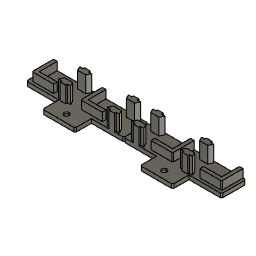
WT#LXLX R+L (Autodesk Fusion 360 design; units mm, degrees)
Autodesk Fusion 360 part; units mm, degrees
note: some values were not read from the file. Set by a fixed rule: which sketch regions a step uses.
sketch "Sketch1" plane through (0, 0, 0) normal (0, 0, 1) x (1, 0, 0)
  line L0 (90, 0) -> (90, 30)
  line L1 (90, 30) -> (0, 30)
  line L2 (0, 30) -> (0, 0)
  line L3 (15, 30) -> (11.5, 30)
  line L4 (15, 30) -> (18.5, 30)
  line L5 (18.5, 30) -> (18.5, 28)
  line L6 (18.5, 28) -> (22.5, 28)
  line L7 (11.5, 30) -> (11.5, 28)
  line L8 (11.5, 28) -> (7.5, 28)
  line L9 (15, 23) -> (20, 23)
  line L10 (15, 23) -> (10, 23)
  line L11 (10, 23) -> (7.5, 28)
  line L12 (20, 23) -> (22.5, 28)
  line L13 (15, 7) -> (10, 7)
  line L14 (15, 7) -> (20, 7)
  line L15 (15, 0) -> (18.5, 0)
  line L16 (18.5, 0) -> (18.5, 2)
  line L17 (18.5, 2) -> (22.5, 2)
  line L18 (22.5, 2) -> (20, 7)
  line L19 (15, 0) -> (11.5, 0)
  line L20 (11.5, 0) -> (11.5, 2)
  line L21 (11.5, 2) -> (7.5, 2)
  line L22 (7.5, 2) -> (10, 7)
  line L23 (75, 30) -> (71.5, 30)
  line L24 (75, 30) -> (78.5, 30)
  line L25 (75, 23) -> (70, 23)
  line L26 (75, 23) -> (80, 23)
  line L27 (78.5, 30) -> (78.5, 28)
  line L28 (78.5, 28) -> (82.5, 28)
  line L29 (82.5, 28) -> (80, 23)
  line L30 (71.5, 30) -> (71.5, 28)
  line L31 (71.5, 28) -> (67.5, 28)
  line L32 (67.5, 28) -> (70, 23)
  line L33 (75, 0) -> (71.5, 0)
  line L34 (75, 7) -> (70, 7)
  line L35 (75, 7) -> (80, 7)
  line L36 (71.5, 0) -> (71.5, 2)
  line L37 (71.5, 2) -> (67.5, 2)
  line L38 (67.5, 2) -> (70, 7)
  line L39 (75, 0) -> (78.5, 0)
  line L40 (78.5, 0) -> (78.5, 2)
  line L41 (78.5, 2) -> (82.5, 2)
  line L42 (82.5, 2) -> (80, 7)
  line L43 (0, 15) -> (30, 15)
  line L44 (30, 30) -> (30, 0)
  line L45 (60, 30) -> (60, 0)
  line L46 (0, 0) -> (30, 0)
  line L47 (30, 0) -> (60, 0)
  line L48 (60, 0) -> (90, 0)
  line L49 (30, 3.5) -> (56.5, 3.5)
  line L50 (56.5, 30) -> (56.5, 3.5)
  line L51 (52, 30) -> (52, 8)
  line L52 (30, 8) -> (52, 8)
  dimension "d1" = 30
  dimension "d2" = 90
  dimension "d8" = 3.5
  dimension "d9" = 7
  dimension "d13" = 7
  dimension "d19" = 4
  dimension "d21" = 3.5
  dimension "d22" = 7
  dimension "d26" = 4
  dimension "d27" = 4
  dimension "d28" = 7
  dimension "d29" = 3.5
  dimension "d35" = 30
  dimension "d38" = 3.5
  dimension "d39" = -8
  constraint vertical L0
  constraint horizontal L1
  constraint vertical L2
  constraint coincident L2.end L46.start
  constraint coincident L1 L3.start
  constraint perpendicular L4 L5
  constraint perpendicular L5 L6
  constraint perpendicular L3 L7
  constraint perpendicular L15 L16
  constraint perpendicular L16 L17
  constraint perpendicular L19 L20
  constraint perpendicular L20 L21
  constraint coincident L1 L23.start
  constraint parallel L1 L24
  constraint perpendicular L1 L27
  constraint perpendicular L27 L28
  constraint perpendicular L1 L30
  constraint perpendicular L30 L31
  constraint perpendicular L36 L37
  constraint perpendicular L39 L40
  constraint perpendicular L40 L41
  constraint midpoint L2 L43.start
  constraint perpendicular L2 L43
  constraint coincident L1 L44.start
  constraint coincident L1 L45.start
  constraint perpendicular L0 L46
  constraint perpendicular L45 L47
  constraint perpendicular L0 L48
  measures "d1" distance of L2.end L1.end
  measures "d2" distance of L2.end L0.start
  measures "d8" distance of L3.start L4.end
  measures "d9" distance of L3.start L9.start
  measures "d13" distance of L15.start L13.start
  measures "d19" distance of L20.end L21.end
  measures "d21" distance of L23.start L24.end
  measures "d22" distance of L23.start L25.start
  measures "d26" distance of L27.end L28.end
  measures "d27" distance of L30.end L31.end
  measures "d28" distance of L33.start L34.start
  measures "d29" distance of L33.start L33.end
  measures "d35" distance of L43.start L43.end
  measures "d59" distance of L2.end
  measures "d63" diameter of L2.end
extrude "Extrude1" add sketch "Sketch1" against normal blind 5 makes body 1
extrude "Extrude2" add sketch "Sketch1" along normal blind 20 contours L33 L34 L35 L36 L37 L38 L39 L40 L41 L42 L48 | L1 L23 L24 L25 L26 L27 L28 L29 L30 L31 L32 | L13 L14 L15 L16 L17 L18 L19 L20 L21 L22 L46 | L1 L3 L4 L5 L6 L7 L8 L9 L10 L11 L12 bodies 1
extrude "Extrude3" add sketch "Sketch1" along normal blind 10 contours L1 L44 L49 L50 L51 L52 bodies 1
chamfer "Chamfer1" distance 1.5 angle 45 4 edges at (90, 0, -2.5) (90, 30, -2.5) (0, 0, -2.5) (0, 30, -2.5) on bodies 1
chamfer "Chamfer2" distance 1 angle 45 1 edges at (56.5, 3.5, 5) on bodies 1
delete_face "DeleteFace1" 1 faces at (89.5, 1, -1.6667) on bodies 1
delete_face "DeleteFace2" 1 faces at (89, 29.5, -3.3333) on bodies 1
extrude "Extrude4" add 1 faces at (90, 10, -1.6667) along direction (1, 0, 0) blind 30 on bodies 1 bodies 1
sketch "Sketch2" plane through (0, 0, 0) normal (0, 0, 1) x (-1, 0, 0)
  line L0 (-120, -30) -> (-78.5, -30)
  line L1 (-78.5, -30) -> (-78.5, -28)
  line L2 (-78.5, -28) -> (-82.5, -28)
  line L3 (-82.5, -28) -> (-80, -23)
  line L4 (-80, -23) -> (-70, -23)
  line L5 (-70, -23) -> (-67.5, -28)
  line L6 (-67.5, -28) -> (-71.5, -28)
  line L7 (-71.5, -28) -> (-71.5, -30)
  line L8 (-71.5, -30) -> (-56.5, -30)
  line L9 (-56.5, -30) -> (-56.5, -4.5)
  line L10 (-56.5, -4.5) -> (-55.5, -3.5)
  line L11 (-55.5, -3.5) -> (-30, -3.5)
  line L12 (-30, -3.5) -> (-30, -8)
  line L13 (-30, -8) -> (-52, -8)
  line L14 (-52, -8) -> (-52, -30)
  line L15 (-52, -30) -> (-18.5, -30)
  line L16 (-18.5, -30) -> (-18.5, -28)
  line L17 (-18.5, -28) -> (-22.5, -28)
  line L18 (-22.5, -28) -> (-20, -23)
  line L19 (-20, -23) -> (-10, -23)
  line L20 (-10, -23) -> (-7.5, -28)
  line L21 (-7.5, -28) -> (-11.5, -28)
  line L22 (-11.5, -28) -> (-11.5, -30)
  line L23 (-11.5, -30) -> (-1.5, -30)
  line L24 (-1.5, -30) -> (0, -28.5)
  line L25 (0, -28.5) -> (0, -1.5)
  line L26 (0, -1.5) -> (-1.5, 0)
  line L27 (-1.5, 0) -> (-11.5, 0)
  line L28 (-11.5, 0) -> (-11.5, -2)
  line L29 (-11.5, -2) -> (-7.5, -2)
  line L30 (-7.5, -2) -> (-10, -7)
  line L31 (-10, -7) -> (-20, -7)
  line L32 (-20, -7) -> (-22.5, -2)
  line L33 (-22.5, -2) -> (-18.5, -2)
  line L34 (-18.5, -2) -> (-18.5, 0)
  line L35 (-18.5, 0) -> (-71.5, 0)
  line L36 (-71.5, 0) -> (-71.5, -2)
  line L37 (-71.5, -2) -> (-67.5, -2)
  line L38 (-67.5, -2) -> (-70, -7)
  line L39 (-70, -7) -> (-80, -7)
  line L40 (-80, -7) -> (-82.5, -2)
  line L41 (-82.5, -2) -> (-78.5, -2)
  line L42 (-78.5, -2) -> (-78.5, 0)
  line L43 (-78.5, 0) -> (-120, 0)
  line L44 (-120, 0) -> (-120, -30)
  line L45 (-120, 0) -> (-90, 0)
  line L46 (-120, 0) -> (-120, -30)
  line L47 (-116.5, -3.5) -> (-90, -3.5)
  line L48 (-116.5, -3.5) -> (-116.5, -30)
  line L49 (-112, -8) -> (-112, -30)
  line L50 (-112, -8) -> (-90, -8)
  line L51 (-90, -3.5) -> (-90, -8)
  dimension "d50" = 30
  dimension "d51" = -3.5
  dimension "d52" = 8
  constraint coincident L43.end L44.start
  constraint perpendicular L44 L45
  constraint coincident L0.start L44.end
  constraint perpendicular L50 L51
  measures "d50" distance of L43.end L45.end
extrude "Extrude5" add sketch "Sketch2" along normal blind 10 contours L0 L47 L48 L49 L50 L51 bodies 1
chamfer "Chamfer3" distance 1 angle 45 1 edges at (116.5, 3.5, 5) on bodies 1
chamfer "Chamfer4" distance 1.5 angle 45 2 edges at (120, 0, -2.5) (120, 30, -2.5) on bodies 1
mirror "Mirror1" about plane through (0, 0, 0) normal (1, 0, 0) of bodies 1 makes body 2
sketch "Sketch3" plane through (0, 0, 0) normal (0, -1, 0) x (1, 0, 0)
  line L0 (-118.5, 0) -> (-118.5, -5)
  line L1 (-118.5, -5) -> (-1.5, -5)
  line L2 (-1.5, -5) -> (-1.5, 0)
  line L3 (-1.5, 0) -> (-11.5, 0)
  line L4 (-11.5, 0) -> (-11.5, 20)
  line L5 (-11.5, 20) -> (-18.5, 20)
  line L6 (-18.5, 20) -> (-18.5, 0)
  line L7 (-18.5, 0) -> (-71.5, 0)
  line L8 (-71.5, 0) -> (-71.5, 20)
  line L9 (-71.5, 20) -> (-78.5, 20)
  line L10 (-78.5, 20) -> (-78.5, 0)
  line L11 (-78.5, 0) -> (-118.5, 0)
  line L12 (-118.5, 0) -> (-1.5, -5)
  line L13 (-60, -2.5) -> (-60, 0)
  line L14 (-60, 0) -> (-80, 0)
  line L15 (-80, 0) -> (-80, -5)
  line L16 (-60, 0) -> (-40, 0)
  line L17 (-40, 0) -> (-40, -5)
  dimension "d59" = 20
  constraint coincident L0.start L11.end
  constraint coincident L1.end L2.start
  constraint midpoint L12 L13.start
  constraint coincident L7 L13.end
  constraint perpendicular L7 L13
  constraint coincident L11 L14.end
  constraint perpendicular L10 L14
  constraint coincident L1 L15.end
  constraint perpendicular L1 L15
  constraint perpendicular L13 L16
  constraint coincident L1 L17.end
  constraint perpendicular L1 L17
  measures "d59" distance of L13.end L16.end
extrude "Extrude6" add sketch "Sketch3" along normal blind 20 contours L7 L11 L12 L13 L14 L15 | L1 L12 L15 L17 | L7 L12 L13 L16 L17 bodies 2
chamfer "Chamfer5" distance 1.5 angle 45 2 edges at (-80, -20, -2.5) (-40, -20, -2.5) on bodies 2
sketch "Sketch4" plane through (0, 0, 0) normal (0, 0, 1) x (-1, 0, 0)
  line L0 (78.5, 0) -> (78.5, -2)
  line L1 (78.5, -2) -> (82.5, -2)
  line L2 (82.5, -2) -> (80, -7)
  line L3 (80, -7) -> (70, -7)
  line L4 (70, -7) -> (67.5, -2)
  line L5 (67.5, -2) -> (71.5, -2)
  line L6 (71.5, -2) -> (71.5, 0)
  line L7 (71.5, 0) -> (78.5, 0)
  line L8 (41.5, 20) -> (40, 18.5)
  line L9 (40, 18.5) -> (40, 0)
  line L10 (40, 0) -> (18.5, 0)
  line L11 (18.5, 0) -> (18.5, -2)
  line L12 (18.5, -2) -> (22.5, -2)
  line L13 (22.5, -2) -> (20, -7)
  line L14 (20, -7) -> (10, -7)
  line L15 (10, -7) -> (7.5, -2)
  line L16 (7.5, -2) -> (11.5, -2)
  line L17 (11.5, -2) -> (11.5, 0)
  line L18 (11.5, 0) -> (1.5, 0)
  line L19 (1.5, 0) -> (0, -1.5)
  line L20 (0, -1.5) -> (0, -28.5)
  line L21 (0, -28.5) -> (1.5, -30)
  line L22 (1.5, -30) -> (11.5, -30)
  line L23 (11.5, -30) -> (11.5, -28)
  line L24 (11.5, -28) -> (7.5, -28)
  line L25 (7.5, -28) -> (10, -23)
  line L26 (10, -23) -> (20, -23)
  line L27 (20, -23) -> (22.5, -28)
  line L28 (22.5, -28) -> (18.5, -28)
  line L29 (18.5, -28) -> (18.5, -30)
  line L30 (18.5, -30) -> (52, -30)
  line L31 (52, -30) -> (52, -8)
  line L32 (52, -8) -> (30, -8)
  line L33 (30, -8) -> (30, -3.5)
  line L34 (30, -3.5) -> (55.5, -3.5)
  line L35 (55.5, -3.5) -> (56.5, -4.5)
  line L36 (56.5, -4.5) -> (56.5, -30)
  line L37 (56.5, -30) -> (71.5, -30)
  line L38 (71.5, -30) -> (71.5, -28)
  line L39 (71.5, -28) -> (67.5, -28)
  line L40 (67.5, -28) -> (70, -23)
  line L41 (70, -23) -> (80, -23)
  line L42 (80, -23) -> (82.5, -28)
  line L43 (82.5, -28) -> (78.5, -28)
  line L44 (78.5, -28) -> (78.5, -30)
  line L45 (78.5, -30) -> (112, -30)
  line L46 (112, -30) -> (112, -8)
  line L47 (112, -8) -> (90, -8)
  line L48 (90, -8) -> (90, -3.5)
  line L49 (90, -3.5) -> (115.5, -3.5)
  line L50 (115.5, -3.5) -> (116.5, -4.5)
  line L51 (116.5, -4.5) -> (116.5, -30)
  line L52 (116.5, -30) -> (118.5, -30)
  line L53 (118.5, -30) -> (120, -28.5)
  line L54 (120, -28.5) -> (120, -1.5)
  line L55 (120, -1.5) -> (118.5, 0)
  line L56 (118.5, 0) -> (80, 0)
  line L57 (80, 0) -> (80, 18.5)
  line L58 (80, 18.5) -> (78.5, 20)
  line L59 (78.5, 20) -> (41.5, 20)
  line L60 (41.5, 20) -> (80, 0)
  line L61 (78.5, 20) -> (40, 0)
  circle A0 centre (60, 10.3896) radius 2.25
  dimension "d63" = 4.5
  constraint coincident L8.start L59.end
  constraint coincident L56.end L57.start
  constraint coincident L58.end L59.start
  constraint coincident L9.end L10.start
  constraint coincident L60 A0.centre
  constraint coincident L61 A0.centre
  measures "d63" diameter of A0
extrude "Extrude7" cut sketch "Sketch4" against normal blind 50 contours L60 L61 A0 | L60 L61 A0 | L60 L61 A0 | L60 L61 A0 bodies 2
chamfer "Chamfer6" distance 1 angle 45 1 edges at (-57.9023, -11.2032, 0) on bodies 2
mirror "Mirror2" about plane through (0, 0, 0) normal (1, 0, 0) of bodies 2 makes body 3
hidden bodies 1
named bodies: "ignore"
